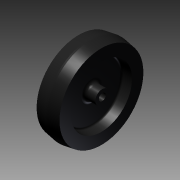
# Autodesk Inventor part: Hjul
Saved by Autodesk Inventor 2012 SP1 (Build 160190100, 190)
## iProperties
Created: 2014-02-18
Part Number: Hjul
Material: Default
Document SubType Name: Modeling
Designer: Pinkponk
Density: 1 g/cm^3
Author: Pinkponk
Autodesk Inventor part; units mm, degrees
ref_plane "YZ Plane" through (0, 0, 0) normal (1, 0, 0) x (0, 1, 0)
ref_plane "XZ Plane" through (0, 0, 0) normal (0, 1, 0) x (-1, 0, 0)
ref_plane "XY Plane" through (0, 0, 0) normal (0, 0, 1) x (1, 0, 0)
sketch "Sketch1" plane through (0, 0, 0) normal (0, 0, 1) x (1, 0, 0)
  line L0 (0, 0) -> (37.6224, 0)
  line L1 (0, 35) -> (0, 48)
  line L2 (0, 48) -> (12.1, 50)
  line L3 (12.1, 50) -> (13.1, 50)
  line L4 (0, 35) -> (11, 34.0376)
  line L5 (11, 34.0376) -> (11, 8)
  line L6 (11, 8) -> (-1, 8)
  line L7 (-1, 8) -> (-1, 0)
  line L8 (13.1, 50) -> (13.1, 0)
  line L9 (-1, 0) -> (13.1, 0)
  line L10 (26.2, 35) -> (26.2, 48)
  line L11 (26.2, 48) -> (14.1, 50)
  line L12 (14.1, 50) -> (13.1, 50)
  line L13 (26.2, 35) -> (15.2, 34.0376)
  line L14 (15.2, 34.0376) -> (15.2, 8)
  line L15 (15.2, 8) -> (27.2, 8)
  line L16 (27.2, 8) -> (27.2, 0)
  line L17 (27.2, 0) -> (13.1, 0)
  point P0 (26.2, 0)
  dimension "d0" = 100
  dimension "d2" = 1
  dimension "d3" = 13
  dimension "d4" = 13.1
  dimension "d5" = 11
  dimension "d6" = 95
  dimension "d7" = 16
  dimension "d8" = 12
  dimension "d9" = 48
  constraints: 36 end point, 8 symmetric about line, 3 perpendicular, 2 point on line, 1 collinear, 1 horizontal, 1 parallel, 1 vertical alignment
  measures "d0" diameter of L3 L0
  measures "d2" distance of L2.end L3.end
  measures "d3" distance of L1.start L1.end
  measures "d4" distance from line of L3.end L1
  measures "d5" distance between parallel lines of L1 L5
  measures "d6" angle of L1 L4
  measures "d7" diameter of L6 L0
  measures "d8" distance between parallel lines of L7 L5
  measures "d9" distance from line of L9 L1.end
revolve "Revolution1" add sketch "Sketch1" angle 360 about axis through (0, 0, 0) along (1, 0, 0)
hole "Hole1" at (27.2, 0, 0) direction (-1, 0, 0) diameter 8 end through all
fillet "Fillet1" radius 4 2 edges at (15.2, -8, 0) (11, -8, 0)
fillet "Fillet2" radius 2 2 edges at (15.2, -34.0376, 0) (11, -34.0376, 0)
body "Solid1"
